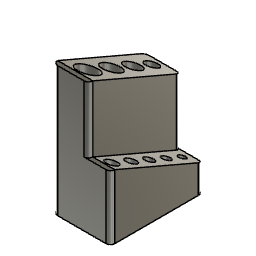
Great Neck Torx Key Holder (Autodesk Fusion 360 design; units mm, degrees)
Autodesk Fusion 360 part; units mm, degrees
sketch "Base Profile" plane through (0, 0, 0) normal (1, 0, 0) x (0, 1, 0)
  line L0 (0, 0) -> (42, 0)
  line L1 (42, 0) -> (42, 42)
  line L2 (42, 42) -> (0, 60)
  line L3 (0, 60) -> (0, 0)
  line L4 (0, 30) -> (42, 12)
  dimension "d1" = 42
  dimension "d2" = 60
  dimension "d3" = 42
  dimension "d4" = 30
  constraint horizontal L0
  constraint vertical L1
  constraint vertical L3
  constraint coincident L0.start L3.end
  constraint coincident L3 L4.start
  constraint coincident L1 L4.end
  constraint parallel L2 L4
  measures "d1" distance of L0.end L1.end
  measures "d2" distance of L0.start L2.end
  measures "d3" distance of L1 L3
  measures "d4" distance of L0.start L4.start
extrude "Extrude1" add sketch "Base Profile" against normal blind 16
extrude "Extrude2" add sketch "Base Profile" along normal blind 10 contours L0 L1 L3 L4
sketch "Hole Layouts" plane through (0, 0, 0) normal (0, 0, 1) x (1, 0, 0)
  line L0 (0, 42) -> (0, 0)
  line L1 (0, 0) -> (10, 0)
  line L2 (10, 0) -> (10, 42)
  line L3 (10, 42) -> (0, 42)
  line L4 (0, 0) -> (0, 42)
  line L5 (0, 42) -> (-16, 42)
  line L6 (-16, 42) -> (-16, 0)
  line L7 (-16, 0) -> (0, 0)
  circle A0 centre (-8, 7.65) radius 4.65
  circle A1 centre (-8, 18.45) radius 4.15
  circle A2 centre (-8, 28.25) radius 3.65
  circle A3 centre (-8, 36.8) radius 2.9
  line L8 (5, 0) -> (5, 42) construction
  circle A4 centre (5, 5.65) radius 2.65
  circle A5 centre (5, 14.4) radius 2.4
  circle A6 centre (5, 22.65) radius 2.15
  circle A7 centre (5, 30.4) radius 1.9
  circle A8 centre (5, 37.65) radius 1.65
  line L9 (-8, 0) -> (-8, 42) construction
  dimension "d10" = 9.3
  dimension "d11" = 8.3
  dimension "d12" = 7.3
  dimension "d13" = 5.8
  dimension "d15" = 2
  dimension "d16" = 2
  dimension "d17" = 2
  dimension "d19" = 3
  dimension "d20" = 2.3
  dimension "d21" = 5.3
  dimension "d22" = 4.8
  dimension "d23" = 4.3
  dimension "d24" = 3.8
  dimension "d25" = 3.3
  dimension "d26" = 3.7
  dimension "d27" = 3.7
  dimension "d29" = 3.7
  dimension "d30" = 3.7
  dimension "d32" = 2.7
  dimension "d33" = 3
  constraint midpoint L1 L8.start
  constraint midpoint L3 L8.end
  constraint coincident L8 A4.centre
  constraint coincident L8 A5.centre
  constraint coincident L8 A6.centre
  constraint coincident L8 A7.centre
  constraint coincident L8 A8.centre
  constraint midpoint L7 L9.start
  constraint midpoint L5 L9.end
  constraint coincident A0.centre L9
  constraint coincident A1.centre L9
  constraint coincident A2.centre L9
  constraint coincident A3.centre L9
  measures "d10" diameter of A0
  measures "d11" diameter of A1
  measures "d12" diameter of A2
  measures "d13" diameter of A3
  measures "d15" distance of A0 A1
  measures "d16" distance of A1 A2
  measures "d17" distance of A2 A3
  measures "d19" distance of L7 A0
  measures "d20" distance of L5 A3
  measures "d21" diameter of A4
  measures "d22" diameter of A5
  measures "d23" diameter of A6
  measures "d24" diameter of A7
  measures "d25" diameter of A8
  measures "d26" distance of A4 A5
  measures "d27" distance of A5 A6
  measures "d29" distance of A6 A7
  measures "d30" distance of A7 A8
  measures "d32" distance of L3 A8
  measures "d33" distance of L1 A4
extrude "Extrude3" cut sketch "Hole Layouts" along normal through all contours A0 | A1 | A2 | A3 | A4 | A5 | A6 | A7 | A8
fillet "Fillet1" radius 2 5 edges at (0, 42, 27) (10, 42, 6) (10, 0, 15) (-16, 42, 21) (-16, 0, 30)
sketch "Clipping corners for Printing" plane through (-16, 0, 0) normal (-1, 0, 0) x (0, -1, 0)
  line L0 (-2, 0) -> (-2, 59.1429)
  line L1 (-2, 59.1429) -> (-40, 42.8571)
  line L2 (-40, 42.8571) -> (-40, 0)
  line L3 (-40, 0) -> (-2, 0)
  line L4 (-42, 42) -> (0, 60)
  line L5 (0, 60) -> (0, 0)
  line L6 (-2, 59.1429) -> (0, 59.1429)
  line L7 (-2, 59.1429) -> (-40, 42.8571)
  line L8 (0, 30) -> (-42, 12)
  line L9 (-2, 0) -> (-2, 29.1429)
  line L10 (-2, 29.1429) -> (0, 29.1429)
  point P0 (-3, 58.7143)
  constraint coincident L4 L0.end
  constraint coincident L5 L6.end
  constraint perpendicular L5 L6
  constraint coincident L0.end L1.start
  constraint coincident L9.end L10.start
  constraint coincident L5 L10.end
  constraint perpendicular L5 L10
extrude "Extrude4" cut sketch "Clipping corners for Printing" against normal through all contours L4 L5 L6
extrude "Extrude5" cut sketch "Clipping corners for Printing" along normal up to surface (10 mm away) from surface at -26 contours L5 L8 L10
fillet "Fillet2" radius 2 1 edges at (0, 0, 44.1429)
equation "d10 = 9 mm + SlipFitTolerance"
equation "d11 = 8 mm + SlipFitTolerance"
equation "d12 = 7 mm + SlipFitTolerance"
equation "d13 = 5.5 mm + SlipFitTolerance"
equation "d16 = d15"
equation "d17 = d15"
equation "d21 = 5 mm + SlipFitTolerance"
equation "d22 = 4.5 mm + SlipFitTolerance"
equation "d23 = 4 mm + SlipFitTolerance"
equation "d24 = 3.5 mm + SlipFitTolerance"
equation "d25 = 3 mm + SlipFitTolerance"
equation "d27 = d26"
equation "d29 = d26"
equation "d30 = d26"
equation "SlipFitTolerance = 0.3 mm"
named bodies: "Torx bit holder"
